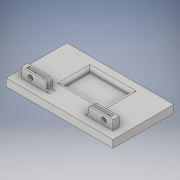
# Autodesk Inventor part: Holder
Saved by Autodesk Inventor 2018 (Build 220112000, 112)
## iProperties
Created: 2019-07-24
Part Number: Holder
Material: Generic
Document SubType Name: Modeling
Designer: Electro707
Density: 1 g/cm^3
Appearance: Default
Description: PCB Holder
Author: Electro707
Autodesk Inventor part; units mm, degrees
ref_plane "YZ Plane" through (0, 0, 0) normal (1, 0, 0) x (0, 1, 0)
ref_plane "XZ Plane" through (0, 0, 0) normal (0, 1, 0) x (-1, 0, 0)
ref_plane "XY Plane" through (0, 0, 0) normal (0, 0, 1) x (1, 0, 0)
sketch "Sketch1" plane through (0, 0, 0) normal (0, 0, 1) x (1, 0, 0)
  circle A0 centre (-24.13, 3.175) radius 1.6
  circle A1 centre (24.13, 3.175) radius 1.6
  line L0 (-30.13, 0) -> (30.13, 0)
  line L1 (30.13, 0) -> (30.13, 6.35)
  line L2 (30.13, 6.35) -> (-30.13, 6.35)
  line L3 (-30.13, 6.35) -> (-30.13, 0)
  line L4 (24.13, 3.175) -> (-24.13, 3.175) construction
  line L5 (-24.13, 3.175) -> (0, 0) construction
  line L6 (0, 0) -> (24.13, 3.175) construction
  line L7 (-30.13, 0) -> (-24.13, 3.175) construction
  line L8 (-30.13, 6.35) -> (-24.13, 3.175) construction
  line L9 (24.13, 3.175) -> (30.13, 6.35) construction
  dimension "d0" = 3.2
  dimension "d1" = 48.26
  dimension "d2" = 6
  dimension "d22" = 6.35
  constraints: 20 end point, 3 equal length, 2 centre point, 2 horizontal, 2 parallel, 1 equal radius, 1 midpoint, 1 perpendicular
  measures "d0" diameter of A0
  measures "d1" distance of L4.start L4.end
  measures "d2" horizontal distance of L4.end L2.end
  measures "d22" distance of L2.end L0.start
extrude "Extrusion1" add sketch "Sketch1" along normal blind 4
sketch "Sketch2" plane through (-30.13, 6.35, 0) normal (0, 1, 0) x (1, 0, 0)
  line L0 (2.19, -3) -> (58.07, -3)
  line L1 (58.07, -3) -> (58.07, -1)
  line L2 (58.07, -1) -> (2.19, -1)
  line L3 (2.19, -1) -> (2.19, -3)
  line L4 (58.07, -1) -> (60.26, 0) construction
  line L5 (0, -4) -> (60.26, -4) construction
  line L6 (58.07, -3) -> (60.26, -4) construction
  line L7 (0, -4) -> (2.19, -3) construction
  point P0 (30.13, 0)
  dimension "d6" = 55.88
  dimension "d7" = 2
  constraints: 14 end point, 2 equal length, 2 parallel, 1 coincident, 1 horizontal, 1 perpendicular
  measures "d6" distance of L1.end L2.end
  measures "d7" distance of L2.end L0.start
extrude "Extrusion2" cut sketch "Sketch2" against normal blind 6.35
sketch "Sketch4" plane through (0, 0, 4) normal (0, 0, 1) x (1, 0, 0)
  line L0 (30.13, 6.35) -> (-30.13, 6.35) projected
  line L1 (-30.13, 0) -> (30.13, 0) projected
  line L2 (-13.75, 6.35) -> (13.75, 6.35)
  line L3 (13.75, 6.35) -> (13.75, 0)
  line L4 (13.75, 0) -> (-13.75, 0)
  line L5 (-13.75, 0) -> (-13.75, 6.35)
  line L6 (13.75, 6.35) -> (0, 0) construction
  line L7 (-13.75, 6.35) -> (0, 0) construction
  dimension "d18" = 27.5
  constraints: 12 end point, 2 parallel, 2 point on line, 1 equal length, 1 horizontal, 1 perpendicular
  measures "d18" distance between parallel lines of L3 L5
extrude "Extrusion4" cut sketch "Sketch4" against normal through all
sketch "Sketch3" plane through (-30.13, 0, 0) normal (0, -1, 0) x (1, 0, 0)
  line L0 (65.26, 9) -> (-5, 9)
  line L1 (-5, 9) -> (-5, -31)
  line L2 (-5, -31) -> (65.26, -31)
  line L3 (65.26, -31) -> (65.26, 9)
  line L4 (0, 4) -> (60.26, 4) construction
  line L5 (0, 4) -> (-5, 9) construction
  line L6 (60.26, 4) -> (65.26, 9) construction
  line L7 (16.88, -6.75) -> (43.38, -6.75)
  line L8 (43.38, -6.75) -> (43.38, -24.25)
  line L9 (43.38, -24.25) -> (16.88, -24.25)
  line L10 (16.88, -24.25) -> (16.88, -6.75)
  line L11 (43.38, -6.75) -> (60.26, 0) construction
  line L12 (43.38, -24.25) -> (65.26, -31) construction
  line L13 (16.88, -6.75) -> (0, 0) construction
  line L14 (16.88, -24.25) -> (-5, -31) construction
  line L15 (16.88, -6.75) -> (16.88, 0) construction
  line L16 (16.88, -24.25) -> (16.88, -31) construction
  line L17 (16.38, 0) -> (0, 0) construction
  point P0 (30.13, 0)
  dimension "d12" = 5
  dimension "d13" = 5
  dimension "d14" = 40
  dimension "d23" = 17.5
  dimension "d24" = 26.5
  constraints: 32 end point, 4 parallel, 3 equal length, 3 perpendicular, 2 horizontal, 2 point on line, 1 vertical
  measures "d12" horizontal distance of L4.start L0.end
  measures "d13" horizontal distance of L4.start L0.end
  measures "d14" distance of L0.end L1.end
  measures "d23" distance of L9.end L7.start
  measures "d24" distance of L8.end L9.end
extrude "Extrusion3" add sketch "Sketch3" along normal blind 5 contours L3 L2 L1 L0 | L7 L8 L9 L10
extrude "Extrusion5" cut sketch "Sketch3" along normal blind 3 contours L7 L8 L9 L10
fillet "Fillet1" radius 2 12 edges at (-13.75, 6.35, 3.5) (-13.75, 6.35, 0.5) (-13.75, 0, 0.5) (-13.75, 0, 3.5) (13.75, 0, 3.5) (13.75, 0, 0.5) (13.75, 6.35, 3.5) (13.75, 6.35, 0.5) (13.25, 0, -15.5) (0, 0, -24.25) (-13.25, 0, -15.5) (0, 0, -6.75)
body "Solid1"
